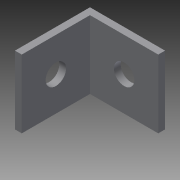
# Autodesk Inventor part: equerre
Saved by Autodesk Inventor 2015 (Build 190159000, 159)
## iProperties
Created: 2015-10-17
Part Number: equerre
Material: Générique
Document SubType Name: Modeling
Designer: astralien3000
Density: 1 g/cm^3
Appearance: Par défaut
Author: astralien3000
Autodesk Inventor part; units mm, degrees
ref_plane "YZ Plane" through (0, 0, 0) normal (1, 0, 0) x (0, 1, 0)
ref_plane "XZ Plane" through (0, 0, 0) normal (0, 1, 0) x (-1, 0, 0)
ref_plane "XY Plane" through (0, 0, 0) normal (0, 0, 1) x (1, 0, 0)
sketch "Esquisse1" plane through (0, 0, 0) normal (0, 0, 1) x (1, 0, 0)
  line L0 (-6, 6) -> (-5, 6)
  line L1 (-5, 6) -> (-5, -5)
  line L2 (-5, -5) -> (-6, -5)
  line L3 (-6, -5) -> (-6, 6)
  line L4 (-5, 6) -> (5, 6)
  line L5 (5, 6) -> (5, 5)
  line L6 (5, 5) -> (-5, 5)
  line L7 (-5, 5) -> (-5, 6)
  point P0 (0, 0)
  dimension "d0" = 1
  dimension "d1" = 1
  dimension "d2" = 10
  dimension "d4" = 5
  dimension "d6" = 10
  dimension "d7" = 5
  constraints: 16 end point, 4 parallel, 2 horizontal, 2 perpendicular, 1 collinear, 1 point on line
  measures "d0" distance of L4.end L5.end
  measures "d1" distance of L1.end L2.end
  measures "d2" distance of L5.end L6.end
  measures "d4" distance from line of L1 point (0, 0)
  measures "d6" distance from line of L2.end L6
  measures "d7" distance from line of L6 point (0, 0)
extrude "Extrusion1" add sketch "Esquisse1" along normal mid plane 10
sketch "Esquisse2" plane through (-5, 5, 5) normal (0, -1, 0) x (1, 0, 0)
  circle A0 centre (5, -5) radius 1.5
  dimension "d10" = 3
  constraints: 1 centre point, 1 coincident
  measures "d10" diameter of A0
extrude "Extrusion2" cut sketch "Esquisse2" against normal through all
sketch "Esquisse3" plane through (-5, -5, 5) normal (1, 0, 0) x (0, 0, -1)
  circle A0 centre (5, 5) radius 1.5
  dimension "d13" = 3
  constraints: 1 centre point, 1 coincident
  measures "d13" diameter of A0
extrude "Extrusion3" cut sketch "Esquisse3" against normal through all
equation "\"d4\" = 0.5 * d2"
equation "\"d7\" = 0.5 * d6"
